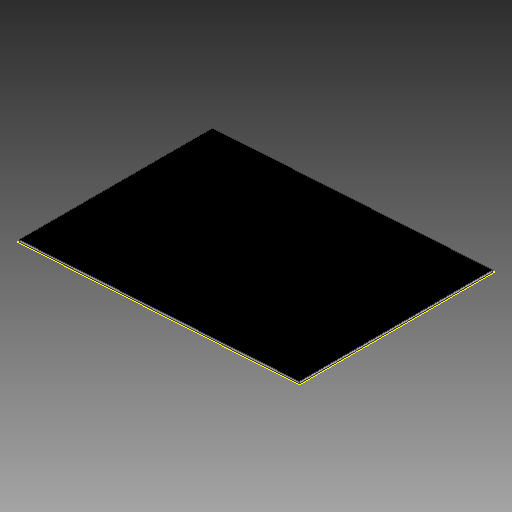
# Autodesk Inventor part: Dach
Saved by Autodesk Inventor 2017 (Build 210142000, 142)
## iProperties
Created: 2017-05-11
Part Number: Dach
Material: Generic
Document SubType Name: Modeling
Designer: Fake
Density: 1 g/cm^3
Appearance: Default
Author: Fake
Autodesk Inventor part; units mm, degrees
ref_plane "YZ Plane" through (0, 0, 0) normal (1, 0, 0) x (0, 1, 0)
ref_plane "XZ Plane" through (0, 0, 0) normal (0, 1, 0) x (-1, 0, 0)
ref_plane "XY Plane" through (0, 0, 0) normal (0, 0, 1) x (1, 0, 0)
ref_plane "Arbeitsebene1" through (3250, -2250, 2500) normal (-0.0614223, 0, 0.9981119) x (0, -1, 0)
sketch "Skizze1" plane through (3250, -2250, 2500) normal (-0.0614223, 0, 0.9981119) x (0, -1, 0)
  line L0 (-100, -100.1892) -> (-4400, -100.1892) projected
  line L1 (-100, -6412.1069) -> (-100, -100.1892) projected
  line L2 (-4400, -6412.1069) -> (-100, -6412.1069) projected
  line L3 (-4400, -100.1892) -> (-4400, -6412.1069) projected
  line L4 (-4500, -6512.2961) -> (-4500, 0) projected
  line L5 (0, -6512.2961) -> (-4500, -6512.2961) projected
  line L6 (0, 0) -> (0, -6512.2961) projected
  line L7 (0, 0) -> (-4500, 0) projected
  line L8 (-4700, -6812.2961) -> (200, -6812.2961)
  line L9 (200, -6812.2961) -> (200, 300)
  line L10 (200, 300) -> (-4700, 300)
  line L11 (-4700, 300) -> (-4700, -6812.2961)
  dimension "d0" = 200
  dimension "d1" = 300
  dimension "d2" = 300
  dimension "d3" = 200
  constraints: 8 end point, 2 parallel, 1 horizontal, 1 perpendicular
  measures "d0" distance between parallel lines of L11 L4
  measures "d1" distance between parallel lines of L7 L10
  measures "d2" distance between parallel lines of L5 L8
  measures "d3" distance between parallel lines of L6 L9
extrude "Extrusion1" add sketch "Skizze1" along normal blind 50 contours L1 L2 L3 L0 | L4 L7 L6 L5 | L11 L10 L9 L8
equation "\"d2\" = d1"
equation "\"d3\" = d0"
